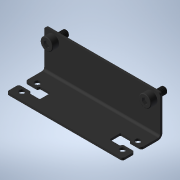
# Autodesk Inventor part: ETH2-14-sensor_plant
Saved by Autodesk Inventor 2021 (Build 250183000, 183)
## iProperties
Created: 2025-05-01
Part Number: ETH2-14-sensor_plant
Material: Generic
Catalog Web Link: www.cadenas.de
Description: GTH4 SENSOR PALNT-GTH4 sensor plant
Vendor: TOYO
Document SubType Name: Modeling
Designer: psAdmin
Manufacturer: TOYO
Mass: 1.89787 g
Surface Area: 38.6127 cm^2
Volume: 1.89787 cm^3
Density: 1 g/cm^3
Appearance: PSOLRGB-175-175-175
Category: PARTsolutions
Company: TOYO
Title: ETH2-14-sensor_plant
Author: Cadenas PARTsolutions
Comments: GTH4 sensor plant
PSOL_IDENT_0: {$CADENAS_DATA/23d-libs/toyo/eth2_series/sensor/eth_sensor_plant.prj},191 {VTYP=3D},{NB=ETH2-14-sens
PSOL_IDENT_1: or_plant},{LINA=ETH2-14-sensor_plant},{NN=GTH4 SENSOR PALNT},{DATE=02.07.2024 05:59:00},{GEOMDATE=27
PSOL_IDENT_2: .06.2024 08:06:59},{VERSION=},{LINEID=10},{WBVAR=},{WBNUMERIC=}  {NB=ETH2-14-sensor_plant},{LINA=ETH
PSOL_IDENT_3: 2-14-sensor_plant},{KT=DUMMY},{IDNR=},{MODEL=ETH2-14}
NB: ETH2-14-sensor_plant
NN: GTH4 SENSOR PALNT
NT: GTH4 sensor plant
NBSYN: $MODEL.-sensor_plant
LINA: ETH2-14-sensor_plant
CATALOG: TOYO
MODEL: ETH2-14
SUPPLIER: TOYO
ARTICLENO: ETH2-14-sensor_plant
BOMINFO: ETH2-14-sensor_plant
CREATOR: CADENAS GmbH
Autodesk Inventor part; units mm, degrees
sketch "Sketch_1" plane through (0, 0, 0) normal (1, 0, 0) x (0, 1, 0)
  line L0 (0, 18) -> (0, 2)
  arc A0 (0, 2) -> (2, 0) centre (2, 2) ccw
  line L1 (2, 0) -> (18, 0)
  line L2 (18, 0) -> (18, 1)
  line L3 (18, 1) -> (2, 1)
  arc A1 (1, 2) -> (2, 1) centre (2, 2) ccw
  line L4 (1, 2) -> (1, 18)
  line L5 (1, 18) -> (0, 18)
  constraints: 12 end point, 4 point on circle, 2 centre point
extrude "Extrusion1" add sketch "Sketch_1" along normal blind 52.5
sketch "Sketch_2" plane through (0, 0, 0) normal (0, 0, 1) x (1, 0, 0)
  arc A0 (1, 18) -> (0, 17) centre (1, 17) ccw
  line L0 (1, 18) -> (51.5, 18)
  arc A1 (52.5, 17) -> (51.5, 18) centre (51.5, 17) ccw
  line L1 (52.5, 17) -> (52.5, 23)
  line L2 (52.5, 23) -> (0, 23)
  line L3 (0, 23) -> (0, 17)
  constraints: 8 end point, 4 point on circle, 2 centre point
extrude "Extrusion2" cut sketch "Sketch_2" along normal blind 1
sketch "Sketch_3" plane through (0, 0, 0) normal (0, 1, 0) x (-1, 0, 0)
  line L0 (5, 0) -> (5, 23)
  line L1 (5, 23) -> (-57.5, 23)
  line L2 (-57.5, 23) -> (-57.5, 0)
  line L3 (-57.5, 0) -> (-52.5, 0)
  line L4 (-52.5, 0) -> (-52.5, 8.5)
  arc A0 (-51.5, 9.5) -> (-52.5, 8.5) centre (-51.5, 8.5) ccw
  line L5 (-51.5, 9.5) -> (-47.5, 9.5)
  arc A1 (-47, 9) -> (-47.5, 9.5) centre (-47.5, 9) ccw
  arc A2 (-47, 9) -> (-46.5, 8.5) centre (-46.5, 9) ccw
  line L6 (-46.5, 8.5) -> (-42.5, 8.5)
  arc A3 (-42.5, 8.5) -> (-42, 9) centre (-42.5, 9) ccw
  line L7 (-42, 9) -> (-42, 13)
  arc A4 (-42, 13) -> (-42.5, 13.5) centre (-42.5, 13) ccw
  line L8 (-42.5, 13.5) -> (-46.5, 13.5)
  arc A5 (-46.5, 13.5) -> (-47, 13) centre (-46.5, 13) ccw
  arc A6 (-47.5, 12.5) -> (-47, 13) centre (-47.5, 13) ccw
  line L9 (-47.5, 12.5) -> (-51.5, 12.5)
  arc A7 (-52.5, 13.5) -> (-51.5, 12.5) centre (-51.5, 13.5) ccw
  line L10 (-52.5, 13.5) -> (-52.5, 17)
  arc A8 (-51.5, 18) -> (-52.5, 17) centre (-51.5, 17) ccw
  line L11 (-51.5, 18) -> (-1, 18)
  arc A9 (0, 17) -> (-1, 18) centre (-1, 17) ccw
  line L12 (0, 17) -> (0, 13.5)
  arc A10 (-1, 12.5) -> (0, 13.5) centre (-1, 13.5) ccw
  line L13 (-1, 12.5) -> (-5, 12.5)
  arc A11 (-5.5, 13) -> (-5, 12.5) centre (-5, 13) ccw
  arc A12 (-5.5, 13) -> (-6, 13.5) centre (-6, 13) ccw
  line L14 (-6, 13.5) -> (-10, 13.5)
  arc A13 (-10, 13.5) -> (-10.5, 13) centre (-10, 13) ccw
  line L15 (-10.5, 13) -> (-10.5, 9)
  arc A14 (-10.5, 9) -> (-10, 8.5) centre (-10, 9) ccw
  line L16 (-10, 8.5) -> (-6, 8.5)
  arc A15 (-6, 8.5) -> (-5.5, 9) centre (-6, 9) ccw
  arc A16 (-5, 9.5) -> (-5.5, 9) centre (-5, 9) ccw
  line L17 (-5, 9.5) -> (-1, 9.5)
  arc A17 (0, 8.5) -> (-1, 9.5) centre (-1, 8.5) ccw
  line L18 (0, 8.5) -> (0, 0)
  line L19 (0, 0) -> (5, 0)
  constraints: 40 end point, 36 point on circle, 18 centre point
extrude "Extrusion3" cut sketch "Sketch_3" along normal blind 1
sketch "Sketch4" plane through (0, 0, 2) normal (0, -1, 0) x (1, 0, 0)
  point P0 (3.5, 5.5)
hole "Hole1" at (3.5, 0, 7.5) direction (0, 1, 0) diameter 2.46 depth 1
pattern_linear "Rectangular Pattern1" count 2 spacing 45.5 along (1, 0, 0) count 2 spacing 7 along (0, 0, 1) of "Hole1"
sketch "Sketch_6" plane through (4, 0, 0) normal (1, 0, 0) x (0, 0, -1)
  line L0 (5, 14.5) -> (-4, 14.5)
  line L1 (-4, 14.5) -> (-4, 16.95)
  arc A0 (-3.7, 17.25) -> (-4, 16.95) centre (-3.7, 16.95) ccw
  line L2 (-3.7, 17.25) -> (-1, 17.25)
  line L3 (-1, 17.25) -> (-1, 16)
  line L4 (-1, 16) -> (4.6935, 16)
  line L5 (4.6935, 16) -> (5, 15.6935)
  line L6 (5, 15.6935) -> (5, 14.5)
  line L7 (5, 14.5) -> (-4, 14.5)
  constraints: 16 end point, 2 point on circle, 1 centre point
revolve "Revolution1" add sketch "Sketch_6" angle 360 about axis through (4, 14.5, -5) along (0, 0, -1)
thread "Thread1" size "M3x0.5" class "6g" standard "ISO Metric profile" length 5.1935
pattern_linear "Rectangular Pattern2" count 2 spacing 44.5 along (1, 0, 0) of "Revolution1"
sketch "Sketch_8" plane through (0, 0, 4) normal (0, 0, 1) x (1, 0, 0)
  line L0 (2.75, 13.7783) -> (4, 13.0566)
  line L1 (4, 13.0566) -> (5.25, 13.7783)
  line L2 (5.25, 13.7783) -> (5.25, 15.2217)
  line L3 (5.25, 15.2217) -> (4, 15.9434)
  line L4 (4, 15.9434) -> (2.75, 15.2217)
  line L5 (2.75, 15.2217) -> (2.75, 13.7783)
  constraints: 12 end point
extrude "Extrusion4" cut sketch "Sketch_8" against normal blind 1.3
pattern_linear "Rectangular Pattern3" count 2 spacing 44.5 along (1, 0, 0) of "Extrusion4"
ref_plane "ip_for_dummy_1_XY" through (0, 14.5, 0) normal (1, 0, 0) x (0, 0, -1)
ref_plane "ip_for_dummy_1_YZ" through (0, 14.5, 0) normal (0, 0, -1) x (0, 1, 0)
ref_plane "ip_for_dummy_1_ZX" through (0, 14.5, 0) normal (0, 1, 0) x (1, 0, 0)
ref_plane "ip_for_dummy_2_XY" through (52.5, 14.5, 0) normal (1, 0, 0) x (0, 0, -1)
ref_plane "ip_for_dummy_2_YZ" through (52.5, 14.5, 0) normal (0, 0, -1) x (0, 1, 0)
ref_plane "ip_for_dummy_2_ZX" through (52.5, 14.5, 0) normal (0, 1, 0) x (1, 0, 0)
ref_plane "ip_for_sensor_1_XY" through (0, 1, 11) normal (1, 0, 0) x (0, 0, -1)
ref_plane "ip_for_sensor_1_YZ" through (0, 1, 11) normal (0, 0, -1) x (0, 1, 0)
ref_plane "ip_for_sensor_1_ZX" through (0, 1, 11) normal (0, 1, 0) x (1, 0, 0)
ref_plane "ip_for_sensor_2_XY" through (52.5, 1, 11) normal (1, 0, 0) x (0, 0, -1)
ref_plane "ip_for_sensor_2_YZ" through (52.5, 1, 11) normal (0, 0, -1) x (0, 1, 0)
ref_plane "ip_for_sensor_2_ZX" through (52.5, 1, 11) normal (0, 1, 0) x (1, 0, 0)
body "Solid1"
